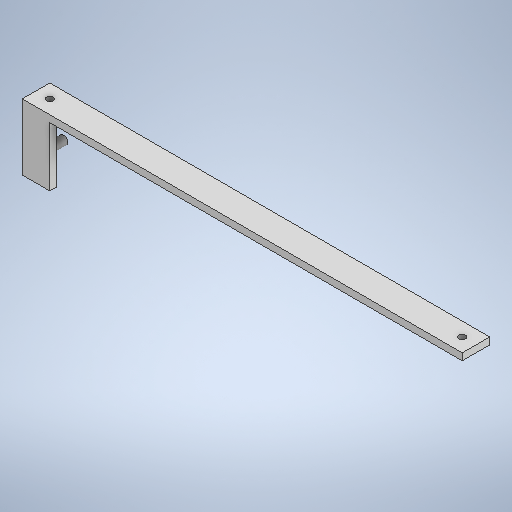
# Autodesk Inventor part: Eje X base - C15
Saved by Autodesk Inventor 2025.3 (Build 293356000, 356)
## iProperties
Created: 2025-11-22
Part Number: Eje X base - C15
Material: Genérico
Document SubType Name: Modeling
Designer: Gianluca Nuñez
Density: 1 g/cm^3
Appearance: Valor por defecto
Author: Gianluca Nuñez
## iProperties of the stored document Ejes Base - C15_3DPrint.ipt
Created: 2025-11-22
Part Number: Ejes Base - C15_3DPrint
Material: Genérico
Document SubType Name: Modeling
Designer: Gianluca Nuñez
Density: 1 g/cm^3
Appearance: Valor por defecto
Author: Gianluca Nuñez
Autodesk Inventor part; units mm, degrees
ref_plane "Plano de trabajo1" through (0, 10, 0) normal (0, 1, 0) x (1, 0, 0)
sketch "Boceto3" plane through (0, 10, 0) normal (0, 1, 0) x (1, 0, 0)
  line L0 (20, -20) -> (0, -20) projected
  line L1 (0, 0) -> (20, 0) projected
  line L2 (0, -20) -> (20, -20)
  line L3 (20, -20) -> (20, 0)
  line L4 (20, 0) -> (0, 0)
  line L5 (0, 0) -> (0, -20)
  constraints: 8 end point, 2 parallel, 1 horizontal, 1 perpendicular
extrude "Extrusión3" add sketch "Boceto3" along normal blind 5
ref_plane "Plano de trabajo4" through (0, -3, 0) normal (0, -1, 0) x (1, 0, 0)
sketch "Boceto8" plane through (0, -3, 0) normal (0, -1, 0) x (1, 0, 0)
  line L0 (0, 0) -> (0, 20) projected
  line L1 (0, 20) -> (20, 20) projected
  line L2 (0, 15) -> (20, 15)
  line L3 (20, 15) -> (20, 20)
  line L4 (20, 20) -> (0, 20)
  line L5 (0, 20) -> (0, 15)
  dimension "d25" = 5
  constraints: 8 end point, 2 parallel, 1 horizontal, 1 perpendicular, 1 point on line
  measures "d25" distance of L2.end L1.end
extrude "Extrusión8" add sketch "Boceto8" along normal blind 30
ref_plane "Plano de trabajo5" through (20, -33, 15) normal (0, 0, -1) x (-1, 0, 0)
sketch "Boceto10" plane through (20, -33, 15) normal (0, 0, -1) x (-1, 0, 0)
  circle A0 centre (10, 17.2) radius 3.15
  line L0 (0, 33) -> (20, 33) projected
  line L1 (0, 32) -> (0, 0) projected
  point P0 (15.75, 33)
  point P1 (10, 33)
  dimension "d35" = 6.3
  dimension "d36" = 15.8
  dimension "d37" = 10
  constraints: 1 centre point, 1 midpoint
  measures "d35" diameter of A0
  measures "d36" distance of point (10, 33) A0.centre
  measures "d37" distance from line of L1 A0.centre
extrude "Extrusión9" add sketch "Boceto10" along normal blind 15
ref_plane "Plano de trabajo2" through (20, 10, 20) normal (1, 0, 0) x (0, 0, -1)
sketch "Boceto13" plane through (0, -3, 0) normal (0, 1, 0) x (1, 0, 0)
  line L0 (0, -20) -> (0, -15) projected
  line L1 (20, -15) -> (20, -20) projected
  line L2 (0, -15) -> (20, -15)
  line L3 (20, -15) -> (20, -20)
  line L4 (20, -20) -> (0, -20)
  line L5 (0, -20) -> (0, -15)
  point P0 (0, 0)
  constraints: 8 end point, 2 parallel, 1 horizontal, 1 perpendicular
extrude "Extrusión12" add sketch "Boceto13" along normal blind 13
sketch "Boceto15" plane through (0, 15, 0) normal (0, 1, 0) x (1, 0, 0)
  circle A0 centre (10, -10) radius 2.5
  line L0 (0, 0) -> (0, -20) projected
  line L1 (0, -20) -> (20, -20) projected
  point P0 (320, -20)
  dimension "d58" = 5
  dimension "d59" = 10
  dimension "d60" = 10
  constraints: 1 centre point
  measures "d58" diameter of A0
  measures "d59" distance from line of L0 A0.centre
  measures "d60" distance from line of L1 A0.centre
extrude "Extrusión14" cut sketch "Boceto15" against normal blind 5
thread "Rosca6" size "M5x0.8" class "6H" standard "ANSI Metric M Profile" full length
sketch "Boceto20" plane through (20, 10, 0) normal (1, 0, 0) x (0, 0, -1)
  line L0 (-20, 5) -> (0, 5) projected
  line L1 (-20, 5) -> (0, 5)
  line L2 (0, 5) -> (0, 0)
  line L3 (0, 0) -> (-20, 0)
  line L4 (-20, 0) -> (-20, 5)
  point P0 (0, -10)
  constraints: 8 end point, 2 parallel, 1 horizontal, 1 perpendicular
extrude "Extrusión18" add sketch "Boceto20" along normal blind 300
sketch "Boceto21" plane through (0, 15, 0) normal (0, 1, 0) x (1, 0, 0)
  circle A0 centre (310, -10) radius 2.5
  line L0 (0, 0) -> (320, 0) projected
  line L1 (320, 0) -> (320, -20) projected
  dimension "d84" = 5
  dimension "d85" = 10
  dimension "d86" = 10
  constraints: 1 centre point
  measures "d84" diameter of A0
  measures "d85" distance from line of L0 A0.centre
  measures "d86" distance from line of L1 A0.centre
extrude "Extrusión19" cut sketch "Boceto21" against normal blind 300
thread "Rosca8" size "M5x0.8" class "6H" standard "ANSI Metric M Profile" full length
